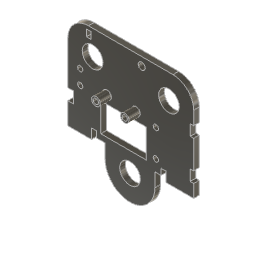
HotendMount (Autodesk Fusion 360 design; units mm, degrees)
Autodesk Fusion 360 part; units mm, degrees
sketch "Sketch1" plane through (0, 0, 0) normal (0, 1, 0) x (1, 0, 0)
  line L0 (0, 0) -> (61, 0)
  line L1 (61, 0) -> (61, -47)
  line L2 (61, -47) -> (0, -47)
  line L3 (0, -47) -> (0, 0)
  circle A0 centre (12, -35) radius 5
  line L4 (0, -16) -> (2.75, -16)
  line L5 (2.75, -16) -> (2.75, -10.55)
  line L6 (2.75, -10.55) -> (0, -10.55)
  line L7 (11.46, 0) -> (11.46, -4.85)
  line L8 (11.46, -4.85) -> (13.91, -4.85)
  line L9 (13.91, -1.85) -> (13.91, -4.85)
  line L10 (18.06, 0) -> (18.06, 4.925)
  line L11 (18.06, 4.925) -> (42.21, 4.925) construction
  line L12 (42.21, 4.925) -> (42.21, 0)
  arc A1 (42.21, 4.925) -> (18.06, 4.925) centre (30.135, 4.925) ccw
  line L13 (45.16, -1.75) -> (45.16, -4.75)
  line L14 (45.16, -4.75) -> (47.61, -4.75)
  line L15 (47.61, -4.75) -> (47.61, 0)
  line L16 (61, -6.3) -> (59.3, -6.3)
  line L17 (59.3, -6.3) -> (59.3, -11.6)
  line L18 (59.3, -11.6) -> (61, -11.6)
  line L19 (61, -25.25) -> (59.3, -25.25)
  line L20 (59.3, -25.25) -> (59.3, -30.55)
  line L21 (59.3, -30.55) -> (61, -30.55)
  line L22 (16, -18.5) -> (38, -18.5)
  line L23 (38, -18.5) -> (38, -4.65)
  line L24 (38, -4.65) -> (16, -4.65)
  line L25 (16, -4.65) -> (16, -18.5)
  circle A2 centre (19.025, -22.5) radius 2.075
  circle A3 centre (33.025, -22.5) radius 2.075
  circle A4 centre (42.7, -20.7) radius 1.5
  circle A5 centre (42.7, -7.4843) radius 1.5
  circle A6 centre (35.8, -43) radius 1.7
  line L26 (13.91, -1.85) -> (18.06, -1.85)
  line L27 (18.06, -1.85) -> (18.06, 0)
  line L28 (30.135, 17) -> (48.0908, 17) construction
  line L29 (42.21, 0) -> (42.21, -1.75)
  line L30 (45.16, -1.75) -> (42.21, -1.75)
  circle A7 centre (49, -35) radius 5
  line L31 (12, -35) -> (49, -35) construction
  line L32 (42.7, -20.7) -> (42.7, -7.4843) construction
  line L33 (9, -45.2) -> (11.2, -45.2)
  line L34 (11.2, -45.2) -> (11.2, -41.9)
  line L35 (11.2, -41.9) -> (9, -41.9)
  line L36 (9, -41.9) -> (9, -45.2)
  line L37 (19.025, -22.5) -> (33.025, -22.5) construction
  circle A8 centre (6, -27) radius 1.5
  circle A9 centre (6, -20) radius 1.5
  line L38 (45.16, 0) -> (45.16, -1.75) construction
  line L39 (13.91, 0) -> (13.91, -1.85) construction
  circle A10 centre (30.135, 4.925) radius 5
  point P0 (6, -27)
  point P1 (6, -20)
  point P2 (12, -35)
  dimension "d1" = 61
  dimension "d2" = 47
  dimension "d3" = 7
  dimension "d4" = 6
  dimension "d5" = 20
  dimension "d20" = 12
  dimension "d21" = 12
  dimension "d22" = 10
  dimension "d25" = 31
  dimension "d26" = 5.45
  dimension "d28" = 2.45
  dimension "d29" = 4.85
  dimension "d30" = 3
  dimension "d32" = 24.15
  dimension "d35" = 11.46
  dimension "d37" = 4.75
  dimension "d38" = 2.45
  dimension "d39" = 13.39
  dimension "d40" = 6.3
  dimension "d41" = 5.3
  dimension "d42" = 1.7
  dimension "d43" = 1.7
  dimension "d44" = 13.65
  dimension "d47" = 5.3
  dimension "d48" = 16.45
  dimension "d49" = 3
  dimension "d50" = 14
  dimension "d51" = 22
  dimension "d52" = 13.85
  dimension "d53" = 16
  dimension "d54" = 4
  dimension "d55" = 10
  dimension "d56" = 12
  dimension "d57" = 25.2
  dimension "d58" = 4
  dimension "d59" = 13.2157
  dimension "d60" = 9
  dimension "d61" = 4.15
  dimension "d62" = 3.4
  dimension "d63" = 3
  dimension "d64" = 3
  dimension "d65" = 6
  dimension "d66" = 20
  dimension "d67" = 3
  dimension "d68" = 18.3
  dimension "d69" = 5.4
  dimension "d70" = 6.6
  dimension "d71" = 26.3
  dimension "d72" = 28.5
  dimension "d73" = 19.025
  dimension "d74" = 10
  dimension "d75" = 3.3
  dimension "d76" = 2.2
  dimension "d77" = 1.8
  dimension "d86" = 2.75
  dimension "d87" = 64
  constraint horizontal L0
  constraint vertical L1
  constraint horizontal L2
  constraint vertical L3
  constraint coincident L0.start L3.end
  constraint vertical P0 P1
  constraint coincident P2 A0.centre
  constraint coincident L3 L4.start
  constraint perpendicular L3 L4
  constraint perpendicular L4 L5
  constraint coincident L3 L6.end
  constraint perpendicular L3 L6
  constraint coincident L0 L7.start
  constraint perpendicular L0 L7
  constraint perpendicular L7 L8
  constraint coincident L0 L39.start
  constraint coincident L0 L10.start
  constraint perpendicular L0 L10
  constraint perpendicular L10 L11
  constraint coincident L0 L12.end
  constraint perpendicular L0 L12
  constraint tangent L12 A1
  constraint coincident L0 L38.start
  constraint perpendicular L0 L13
  constraint perpendicular L13 L14
  constraint coincident L0 L15.end
  constraint perpendicular L0 L15
  constraint perpendicular L8 L9
  constraint coincident L1 L16.start
  constraint perpendicular L1 L16
  constraint perpendicular L16 L17
  constraint perpendicular L1 L18
  constraint coincident L1 L19.start
  constraint perpendicular L1 L19
  constraint perpendicular L19 L20
  constraint coincident L1 L21.end
  constraint perpendicular L1 L21
  constraint horizontal L22
  constraint vertical L23
  constraint horizontal L24
  constraint vertical L25
  constraint perpendicular L9 L26
  constraint vertical L27
  constraint midpoint A1 L28.start
  constraint tangent A1 L28
  constraint horizontal L28
  constraint coincident L1 L18.end
  constraint perpendicular L0 L29
  constraint horizontal L30
  constraint equal A2 A3
  constraint coincident A7.centre L31.end
  constraint horizontal L31
  constraint coincident A4.centre L32.start
  constraint coincident A5.centre L32.end
  constraint vertical L32
  constraint horizontal L33
  constraint vertical L34
  constraint horizontal L35
  constraint vertical L36
  constraint coincident A2.centre L37.start
  constraint coincident A3.centre L37.end
  constraint horizontal L37
  constraint equal A4 A5
  constraint coincident P0 A8.centre
  constraint coincident P1 A9.centre
  constraint perpendicular L0 L38
  constraint perpendicular L8 L39
  constraint concentric A1 A10
  measures "d1" distance of L0.start L0.end
  measures "d2" distance of L0.start L2.end
  measures "d3" distance of P0 P1
  measures "d4" distance of L3 P1
  measures "d5" distance of L2 P0
  measures "d20" distance of L2 P2
  measures "d21" distance of L3 P2
  measures "d22" diameter of A0
  measures "d25" distance of L2 L4
  measures "d26" distance of L4.end L5.end
  measures "d28" distance of L7.end L8.end
  measures "d29" distance of L7.start L7.end
  measures "d30" distance of L8 L26
  measures "d32" distance of L10 L12
  measures "d35" distance of L3 L7
  measures "d37" distance of L14.end L15.end
  measures "d38" distance of L13.end L14.end
  measures "d39" distance of L1 L15
  measures "d40" distance of L0 L16
  measures "d41" distance of L16.end L17.end
  measures "d42" distance of L17.end L18.end
  measures "d43" distance of L19.start L19.end
  measures "d44" distance of L18.end L19.start
  measures "d47" distance of L19.end L20.end
  measures "d48" distance of L1.end L21.end
  measures "d49" distance of L14 L30
  measures "d50" distance of A2.centre A3.centre
  measures "d51" distance of L22.start L22.end
  measures "d52" distance of L22.start L24.end
  measures "d53" distance of L3 L25
  measures "d54" distance of L22 A3.centre
  measures "d55" diameter of A7
  measures "d56" distance of L1 A7.centre
  measures "d57" distance of L1 A6.centre
  measures "d58" distance of L2 A6.centre
  measures "d59" distance of A4.centre A5.centre
  measures "d60" distance of L3 L36
  measures "d61" diameter of A3
  measures "d62" diameter of A6
  measures "d63" diameter of A4
  measures "d64" diameter of A8
  measures "d65" distance of L3 P0
  measures "d66" distance of L2 P0
  measures "d67" diameter of A9
  measures "d68" distance of L1 A4.centre
  measures "d69" distance of L12 L15
  measures "d70" distance of L7 L27
  measures "d71" distance of L2 A4.centre
  measures "d72" distance of L2 L22
  measures "d73" distance of L3 A2.centre
  measures "d74" diameter of A10
  measures "d75" distance of L33.end L34.end
  measures "d76" distance of L33.start L33.end
  measures "d77" distance of L2 L33
  measures "d86" distance of L5.end L6.end
  measures "d87" distance of L2 L28
extrude "Extrude1" add sketch "Sketch1" along normal blind 2.75 contours L0 L1 L2 L3 L4 L5 L6 L7 L8 L9 L13 L14 L15 L16 L17 L18 L19 L20 L21 L26 L27 L29 L30 A10 | L0 L10 L12 A1 A10 | A2 | A3
extrude "Extrude3" add sketch "Sketch1" against normal blind 5.42 contours A2 | A3
fillet "Fillet1" radius 10 2 edges at (0, 1.375, 47) (61, 1.375, 47)
hole "Hole3" at (19.025, -5.42, 22.5) direction (0, 1, 0) diameter 3 end through all
hole "Hole4" at (33.025, -5.42, 22.5) direction (0, 1, 0) diameter 3 depth 8.17 tip angle 118
thread "Thread1" "ISO Metric profile 3.0 M3x0.5 6H" major diameter 3.086 minor diameter 2.529 pitch 0.5 angle 60 resizes the face on face at (43.1777, 1.8333, 19.2781)
thread "Thread2" "ISO Metric profile 3.0 M3x0.5 6H" major diameter 3.086 minor diameter 2.529 pitch 0.5 angle 60 resizes the face on face at (43.1063, 1.8333, 8.9282)
thread "Thread3" "ISO Metric profile 3.0 M3x0.5 6H" major diameter 3.086 minor diameter 2.529 pitch 0.5 angle 60 resizes the face on face at (19.1744, -2.6967, 23.9925)
thread "Thread4" "ISO Metric profile 3.0 M3x0.5 6H" major diameter 3.086 minor diameter 2.529 pitch 0.5 angle 60 resizes the face on face at (33.538, -2.6967, 21.0905)
thread "Thread5" "ISO Metric profile 3.0 M3x0.5 6H" major diameter 3.086 minor diameter 2.529 pitch 0.5 angle 60 resizes the face on face at (7.4925, 1.8333, 19.8506)
thread "Thread6" "ISO Metric profile 3.0 M3x0.5 6H" major diameter 3.086 minor diameter 2.529 pitch 0.5 angle 60 resizes the face on face at (7.4925, 1.8333, 26.8506)
extrude "Extrude2" [suppressed]
equation "d71 = 24.8 mm + ( d63 / 2 )"
equation "d73 = 21.1 mm - d61 / 2"
